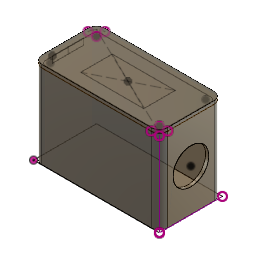
box (Autodesk Fusion 360 design; units mm, degrees)
Autodesk Fusion 360 part; units mm, degrees
sketch "Base" plane through (0, 0, 0) normal (0, 1, 0) x (1, 0, 0) in component "Top"
  line L0 (0, 0) -> (60, 0)
  line L1 (60, 0) -> (60, 30)
  line L2 (60, 30) -> (0, 30)
  line L3 (0, 30) -> (0, 0)
  dimension "d6" = 60
  dimension "d7" = 30
  measures "d6" distance of L0.start
  measures "d7" distance of L0.start
extrude "Extrude1" add sketch "Base" along normal blind 40 makes body 1 in component "Top"
fillet "Fillet1" radius 4 4 edges at (60, 20, 0) (0, 20, 0) (60, 20, -30) (0, 20, -30) on bodies 1 in component "Top"
shell "Shell1" thickness 1.5 removed faces 1 at (38.6667, 40, -10) on bodies 1 in component "Top"
sketch "Knob" plane through (1.5, 0, 0) normal (1, 0, 0) x (0, 0, -1) in component "Top"
  line L0 (26, 1.5) -> (26, 40)
  line L1 (26, 40) -> (4, 40)
  line L2 (4, 40) -> (4, 1.5)
  line L3 (4, 1.5) -> (26, 1.5)
  line L4 (7.5, 40) -> (22.5, 40)
  line L5 (22.5, 40) -> (22.5, 37)
  line L6 (22.5, 37) -> (7.5, 37)
  line L7 (7.5, 37) -> (7.5, 40)
  line L8 (15, 40) -> (15, 37) construction
  dimension "d12" = 15
  dimension "d13" = 3
  measures "d12" distance of origin
extrude "Extrude2" add sketch "Knob" along normal blind 6 draft -45 contours L1 L4 L5 L6 L7 bodies 1 in component "Top"
ref_plane "WorkPlane2" through (30, 20, -15) normal (-1, 0, 0) x (0, 0, 1) in component "Top"
mirror "Mirror1" about plane through (30, 20, -15) normal (-1, 0, 0) of "Extrude2" in component "Top"
sketch "Top" plane through (0, 40, 0) normal (0, 1, 0) x (-1, 0, 0) in component "Base"
  line L0 (-60, -4) -> (-60, -26)
  arc A0 (-60, -26) -> (-56, -30) centre (-56, -26) ccw
  line L1 (-56, -30) -> (-4, -30)
  arc A1 (-4, -30) -> (0, -26) centre (-4, -26) ccw
  line L2 (0, -26) -> (0, -4)
  arc A2 (0, -4) -> (-4, 0) centre (-4, -4) ccw
  line L3 (-4, 0) -> (-56, 0)
  arc A3 (-56, 0) -> (-60, -4) centre (-56, -4) ccw
  line L4 (-58.5, -7.5) -> (-58.5, -4)
  arc A4 (-56, -1.5) -> (-58.5, -4) centre (-56, -4) ccw
  line L5 (-56, -1.5) -> (-4, -1.5)
  arc A5 (-1.5, -4) -> (-4, -1.5) centre (-4, -4) ccw
  line L6 (-1.5, -4) -> (-1.5, -7.5)
  line L7 (-1.5, -7.5) -> (-1.5, -22.5)
  line L8 (-1.5, -22.5) -> (-1.5, -26)
  arc A6 (-4, -28.5) -> (-1.5, -26) centre (-4, -26) ccw
  line L9 (-4, -28.5) -> (-56, -28.5)
  arc A7 (-58.5, -26) -> (-56, -28.5) centre (-56, -26) ccw
  line L10 (-58.5, -26) -> (-58.5, -22.5)
  line L11 (-58.5, -22.5) -> (-58.5, -7.5)
extrude "Extrude1'" add sketch "Top" along normal blind 1.5 separate body contours L0 A0 L1 A1 L2 A2 L3 A3 | L4 A4 L5 A5 L6 L7 L8 A6 L9 A7 L10 L11 makes body 2 in component "Base"
sketch "Lip" plane through (0, 40, 0) normal (0, -1, 0) x (1, 0, 0) in component "Base"
  arc A0 (60, -4) -> (56, 0) centre (56, -4) ccw
  line L0 (56, 0) -> (4, 0)
  arc A1 (4, 0) -> (0, -4) centre (4, -4) ccw
  line L1 (0, -4) -> (0, -26)
  arc A2 (0, -26) -> (4, -30) centre (4, -26) ccw
  line L2 (4, -30) -> (56, -30)
  arc A3 (56, -30) -> (60, -26) centre (56, -26) ccw
  line L3 (60, -26) -> (60, -4)
  line L4 (58.3, -26) -> (58.3, -4)
  arc A4 (58.3, -4) -> (56, -1.7) centre (56, -4) ccw
  line L5 (56, -1.7) -> (4, -1.7)
  arc A5 (4, -1.7) -> (1.7, -4) centre (4, -4) ccw
  line L6 (1.7, -4) -> (1.7, -26)
  arc A6 (1.7, -26) -> (4, -28.3) centre (4, -26) ccw
  line L7 (4, -28.3) -> (56, -28.3)
  arc A7 (56, -28.3) -> (58.3, -26) centre (56, -26) ccw
  dimension "d19" = 1.7
  measures "d19" distance of L3
extrude "Extrude2'" add sketch "Lip" along normal blind 3 contours L4 A4 L5 A5 L6 A6 L7 A7 bodies 2 in component "Base"
extrude "Extrude3" cut sketch "Knob" along normal blind 3 draft -45 from surface at 0.2 contours L1 L4 L5 L6 L7 bodies 2 in component "Base"
mirror "Mirror1'" about plane through (30, 20, -15) normal (-1, 0, 0) of "Extrude3" in component "Base"
shell "Shell1'" thickness 1.5 removed faces 1 at (38.6667, 37, -10.5667) on bodies 2 in component "Base"
chamfer "Chamfer1" distance 0.6 angle 45 2 edges at (1.7, 37, -15) (58.3, 37, -15) on bodies 2 in component "Base"
sketch "PCB Mount" plane through (0, 40, 0) normal (0, -1, 0) x (1, 0, 0) in component "Base"
  arc A0 (60, -4) -> (56, 0) centre (56, -4) ccw construction
  arc A1 (0, -26) -> (4, -30) centre (4, -26) ccw construction
  line L0 (58.8284, -1.1716) -> (1.1716, -28.8284) construction
  line L1 (45, -22.5) -> (15, -22.5)
  line L2 (15, -22.5) -> (15, -7.5)
  line L3 (15, -7.5) -> (45, -7.5)
  line L4 (45, -7.5) -> (45, -22.5)
  line L5 (45, -22.5) -> (15, -7.5) construction
  line L6 (15, -22.5) -> (45, -7.5) construction
  dimension "d33" = 30
  dimension "d34" = 15
extrude "Extrude5" add sketch "PCB Mount" along normal blind 3 bodies 2 in component "Base"
sketch "Right Holes" plane through (60, 0, 0) normal (1, 0, 0) x (0, 0, -1) in component "Top"
  line L0 (26, 40) -> (4, 40)
  line L1 (4, 40) -> (4, 0)
  line L2 (4, 0) -> (26, 0)
  line L3 (26, 0) -> (26, 40)
  circle A0 centre (15, 20) radius 8.5
  line L4 (0, 40) -> (0, 0)
  line L5 (0, 0) -> (30, 0)
  dimension "d41" = 17
  dimension "d42" = 15
  dimension "d43" = 20
  measures "d41" diameter of A0
  measures "d42" distance of L4
  measures "d43" distance of L5
extrude "Extrude3'" cut sketch "Right Holes" against normal up to surface (1.5 mm away) contours A0 bodies 1 in component "Top"
extrude "Extrude4" [suppressed] in component "Top"
component "Enclosure" placed x (1, 0, 0) y (0, 1, 0) z (0, 0, 1) at (0, 0, 0)
component "Top" placed x (1, 0, 0) y (0, 1, 0) z (0, 0, 1) at (0, 0, 0) in component "Enclosure"
component "Base" placed x (1, 0, 0) y (0, 1, 0) z (0, 0, 1) at (0, 0, 0) in component "Enclosure"
equation "Width = 30 mm"
equation "length = 60 mm"
equation "heigth = 40 mm"
equation "shell = 1.5 mm"
equation "gap = 0.2 mm"
equation "d6 = length"
equation "d7 = Width"
equation "d8 = heigth"
equation "d11 = shell"
equation "d12 = Width / 2"
equation "d13 = shell * 2"
equation "d17 = shell"
equation "d19 = shell + gap"
equation "d20 = shell * 2"
equation "d23 = shell * 2"
equation "d26 = shell"
equation "d33 = length / 2"
equation "d34 = Width / 2"
equation "d42 = Width / 2"
equation "d43 = heigth / 2"
